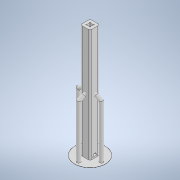
# Autodesk Inventor part: 130mm Rod Template
Saved by Autodesk Inventor 2022 (Build 260153000, 153)
## iProperties
Created: 2022-06-07
Part Number: 130mm Rod Template
Material: Generic
Document SubType Name: Modeling
Designer: Nick
Density: 1 g/cm^3
Appearance: Default
Author: Nick
Autodesk Inventor part; units mm, degrees
ref_plane "YZ Plane" through (0, 0, 0) normal (1, 0, 0) x (0, 1, 0)
ref_plane "XZ Plane" through (0, 0, 0) normal (0, 1, 0) x (-1, 0, 0)
ref_plane "XY Plane" through (0, 0, 0) normal (0, 0, 1) x (1, 0, 0)
sketch "Sketch1" plane through (0, 0, 0) normal (0, 1, 0) x (-1, 0, 0)
  circle A0 centre (0, 0) radius 2
  arc A1 (2.5, 2.179449) -> (2.5, -2.179449) centre (7, 0) ccw
  arc A2 (2.179449, -2.5) -> (-2.179449, -2.5) centre (0, -7) ccw
  arc A3 (-2.5, -2.179449) -> (-2.5, 2.179449) centre (-7, 0) ccw
  arc A4 (-2.179449, 2.5) -> (2.179449, 2.5) centre (0, 7) ccw
  line L0 (2.5, 2.5) -> (-2.5, 2.5)
  line L1 (-2.5, 2.5) -> (-2.5, -2.5)
  line L2 (-2.5, -2.5) -> (2.5, -2.5)
  line L3 (2.5, -2.5) -> (2.5, 2.5)
  line L4 (-5.5, -5.5) -> (-5.5, 5.5)
  line L5 (-5.5, 5.5) -> (5.5, 5.5)
  line L6 (5.5, 5.5) -> (5.5, -5.5)
  line L7 (5.5, -5.5) -> (-5.5, -5.5)
  point P0 (2.5, 0)
  point P1 (0, -2.5)
  dimension "d0" = 4
  dimension "d1" = 5
  dimension "d2" = 5
  dimension "d3" = 3
  constraints: 16 end point, 8 point on circle, 8 point on line, 5 centre point, 4 parallel, 4 tangent, 3 equal radius, 3 horizontal alignment, 3 perpendicular, 3 vertical alignment, 2 midpoint, 1 coincident, 1 horizontal, 3 other
  measures "d0" diameter of A0
  measures "d1" distance of L0.start L0.end
  measures "d2" radius of A4
  measures "d3" distance between parallel lines of L1 L4
extrude "Extrusion1" add sketch "Sketch1" along normal blind 127 contours A1 L3 | A4 L0 | A2 L2 | A3 L1 | L4 L5 L6 L7
sketch "Sketch2" plane through (5.5, 0, -5.5) normal (0, 0, -1) x (-1, 0, 0)
  line L0 (11, 127) -> (11, 0) construction
  line L1 (11, 0) -> (0, 0) construction
  line L2 (0, 0) -> (0, 127) construction
  line L3 (0, 127) -> (11, 127) construction
  line L4 (0, 0) -> (0, 127)
  line L5 (0, 127) -> (11, 127)
  line L6 (11, 0) -> (11, 127)
  line L7 (0, 0) -> (11, 0)
  line L8 (2.45, 73.51013) -> (2.45, 76.485981)
  line L9 (2.45, 76.485981) -> (3.072853, 76.485981)
  line L10 (3.072853, 76.485981) -> (3.072853, 75.378688)
  line L11 (3.072853, 75.378688) -> (7.16094, 75.378688)
  line L12 (7.16094, 75.378688) -> (7.16094, 76.485981)
  line L13 (7.16094, 76.485981) -> (7.71953, 76.485981)
  spline S0 degree 2 poles (7.71953, 76.485981) (7.71953, 75.858185) (8.075446, 75.264993) (8.569773, 75.225446) knots 0 0 0 1 2 2 2
  line L14 (8.569773, 75.225446) -> (8.569773, 74.592707)
  line L15 (8.569773, 74.592707) -> (3.072853, 74.592707)
  line L16 (3.072853, 74.592707) -> (3.072853, 73.51013)
  line L17 (3.072853, 73.51013) -> (2.45, 73.51013)
  spline S1 degree 2 poles (7.971637, 70.741897) (7.971637, 70.964344) (7.862885, 71.404296) (7.778849, 71.616856) knots 0 0 0 1 2 2 2
  spline S2 degree 2 poles (7.778849, 71.616856) (7.694814, 71.814587) (7.516856, 72.10624) (7.437764, 72.219936) knots 0 0 0 1 2 2 2
  line L18 (7.437764, 72.219936) -> (7.437764, 72.269368)
  line L19 (7.437764, 72.269368) -> (8.302836, 72.269368)
  spline S3 degree 2 poles (8.302836, 72.269368) (8.446191, 72.002432) (8.678525, 71.087926) (8.678525, 70.677634) knots 0 0 0 1 2 2 2
  spline S4 degree 2 poles (8.678525, 70.677634) (8.678525, 70.262399) (8.510454, 69.64449) (8.332496, 69.392383) knots 0 0 0 1 2 2 2
  spline S5 degree 2 poles (8.332496, 69.392383) (8.139708, 69.125446) (7.581118, 68.848623) (7.20543, 68.848623) knots 0 0 0 1 2 2 2
  spline S6 degree 2 poles (7.20543, 68.848623) (6.701216, 68.848623) (5.939951, 69.511022) (5.841086, 69.975689) knots 0 0 0 1 2 2 2
  line L20 (5.841086, 69.975689) -> (5.781767, 69.975689)
  spline S7 degree 2 poles (5.781767, 69.975689) (5.742221, 69.782902) (5.564263, 69.34295) (5.386305, 69.155106) knots 0 0 0 1 2 2 2
  spline S8 degree 2 poles (5.386305, 69.155106) (5.21329, 68.967261) (4.659644, 68.729984) (4.259238, 68.729984) knots 0 0 0 1 2 2 2
  spline S9 degree 2 poles (4.259238, 68.729984) (3.848947, 68.729984) (3.151945, 69.011751) (2.885008, 69.268801) knots 0 0 0 1 2 2 2
  spline S10 degree 2 poles (2.885008, 69.268801) (2.608185, 69.535738) (2.321475, 70.292059) (2.321475, 70.771556) knots 0 0 0 1 2 2 2
  spline S11 degree 2 poles (2.321475, 70.771556) (2.321475, 71.231281) (2.543922, 72.130957) (2.697164, 72.43744) knots 0 0 0 1 2 2 2
  line L21 (2.697164, 72.43744) -> (3.562237, 72.43744)
  line L22 (3.562237, 72.43744) -> (3.562237, 72.37812)
  spline S12 degree 2 poles (3.562237, 72.37812) (3.374392, 72.12107) (3.028363, 71.251054) (3.028363, 70.820989) knots 0 0 0 1 2 2 2
  spline S13 degree 2 poles (3.028363, 70.820989) (3.028363, 70.568882) (3.186548, 70.064668) (3.369449, 69.896597) knots 0 0 0 1 2 2 2
  spline S14 degree 2 poles (3.369449, 69.896597) (3.55235, 69.733469) (3.987358, 69.560454) (4.318558, 69.560454) knots 0 0 0 1 2 2 2
  spline S15 degree 2 poles (4.318558, 69.560454) (4.649757, 69.560454) (5.079822, 69.753242) (5.203404, 69.926257) knots 0 0 0 1 2 2 2
  spline S16 degree 2 poles (5.203404, 69.926257) (5.326986, 70.099271) (5.420908, 70.568882) (5.420908, 70.845706) knots 0 0 0 1 2 2 2
  line L23 (5.420908, 70.845706) -> (5.420908, 71.191735)
  line L24 (5.420908, 71.191735) -> (6.098136, 71.191735)
  line L25 (6.098136, 71.191735) -> (6.098136, 70.919855)
  spline S17 degree 2 poles (6.098136, 70.919855) (6.098136, 70.371151) (6.622123, 69.679093) (7.121394, 69.679093) knots 0 0 0 1 2 2 2
  spline S18 degree 2 poles (7.121394, 69.679093) (7.353728, 69.679093) (7.684927, 69.857051) (7.783793, 70.000406) knots 0 0 0 1 2 2 2
  spline S19 degree 2 poles (7.783793, 70.000406) (7.887601, 70.153647) (7.971637, 70.529336) (7.971637, 70.741897) knots 0 0 0 1 2 2 2
  spline S20 degree 2 poles (5.5, 64.014101) (3.858833, 64.014101) (2.321475, 64.968153) (2.321475, 65.961751) knots 0 0 0 1 2 2 2
  spline S21 degree 2 poles (2.321475, 65.961751) (2.321475, 66.970179) (3.888493, 67.914344) (5.495057, 67.914344) knots 0 0 0 1 2 2 2
  spline S22 degree 2 poles (5.495057, 67.914344) (7.14611, 67.914344) (8.673582, 66.960292) (8.673582, 65.961751) knots 0 0 0 1 2 2 2
  spline S23 degree 2 poles (8.673582, 65.961751) (8.673582, 64.958266) (7.091734, 64.014101) (5.5, 64.014101) knots 0 0 0 1 2 2 2
  spline S24 degree 2 poles (3.641329, 65.062075) (3.942869, 64.943436) (4.872204, 64.844571) (5.5, 64.844571) knots 0 0 0 1 2 2 2
  spline S25 degree 2 poles (5.5, 64.844571) (6.127796, 64.844571) (7.052188, 64.943436) (7.363614, 65.067018) knots 0 0 0 1 2 2 2
  spline S26 degree 2 poles (7.363614, 65.067018) (7.675041, 65.1906) (7.996353, 65.620665) (7.996353, 65.961751) knots 0 0 0 1 2 2 2
  spline S27 degree 2 poles (7.996353, 65.961751) (7.996353, 66.302837) (7.675041, 66.742788) (7.353728, 66.871313) knots 0 0 0 1 2 2 2
  spline S28 degree 2 poles (7.353728, 66.871313) (7.042302, 66.994895) (6.093193, 67.083874) (5.495057, 67.083874) knots 0 0 0 1 2 2 2
  spline S29 degree 2 poles (5.495057, 67.083874) (4.852431, 67.083874) (3.992302, 67.004782) (3.656159, 66.876257) knots 0 0 0 1 2 2 2
  spline S30 degree 2 poles (3.656159, 66.876257) (3.339789, 66.757618) (2.998703, 66.317667) (2.998703, 65.961751) knots 0 0 0 1 2 2 2
  spline S31 degree 2 poles (2.998703, 65.961751) (2.998703, 65.625608) (3.320016, 65.185657) (3.641329, 65.062075) knots 0 0 0 1 2 2 2
  line L26 (2.45, 57.928931) -> (5.099595, 57.928931)
  spline S32 degree 2 poles (5.099595, 57.928931) (5.415964, 57.928931) (5.954781, 57.978363) (6.10308, 58.057456) knots 0 0 0 1 2 2 2
  spline S33 degree 2 poles (6.10308, 58.057456) (6.266208, 58.136548) (6.424392, 58.438088) (6.424392, 58.700081) knots 0 0 0 1 2 2 2
  spline S34 degree 2 poles (6.424392, 58.700081) (6.424392, 58.937358) (6.132739, 59.481119) (5.855916, 59.767828) knots 0 0 0 1 2 2 2
  spline S35 degree 2 poles (5.855916, 59.767828) (5.78671, 59.762885) (5.593922, 59.752999) (5.465397, 59.752999) knots 0 0 0 1 2 2 2
  line L27 (5.465397, 59.752999) -> (2.45, 59.752999)
  line L28 (2.45, 59.752999) -> (2.45, 60.524149)
  line L29 (2.45, 60.524149) -> (5.099595, 60.524149)
  spline S36 degree 2 poles (5.099595, 60.524149) (5.415964, 60.524149) (5.954781, 60.573582) (6.10308, 60.652675) knots 0 0 0 1 2 2 2
  spline S37 degree 2 poles (6.10308, 60.652675) (6.266208, 60.731767) (6.424392, 61.033307) (6.424392, 61.2953) knots 0 0 0 1 2 2 2
  spline S38 degree 2 poles (6.424392, 61.2953) (6.424392, 61.542464) (6.112966, 62.091167) (5.870746, 62.348218) knots 0 0 0 1 2 2 2
  line L30 (5.870746, 62.348218) -> (2.45, 62.348218)
  line L31 (2.45, 62.348218) -> (2.45, 63.119368)
  line L32 (2.45, 63.119368) -> (7.027472, 63.119368)
  line L33 (7.027472, 63.119368) -> (7.027472, 62.348218)
  line L34 (7.027472, 62.348218) -> (6.523258, 62.348218)
  spline S39 degree 2 poles (6.523258, 62.348218) (6.824798, 62.046678) (7.155997, 61.453485) (7.155997, 61.097569) knots 0 0 0 1 2 2 2
  spline S40 degree 2 poles (7.155997, 61.097569) (7.155997, 60.692221) (6.785251, 60.064425) (6.365073, 59.901297) knots 0 0 0 1 2 2 2
  spline S41 degree 2 poles (6.365073, 59.901297) (6.755592, 59.550324) (7.155997, 58.887926) (7.155997, 58.50235) knots 0 0 0 1 2 2 2
  spline S42 degree 2 poles (7.155997, 58.50235) (7.155997, 58.205754) (6.973096, 57.721313) (6.765478, 57.543355) knots 0 0 0 1 2 2 2
  spline S43 degree 2 poles (6.765478, 57.543355) (6.557861, 57.360454) (5.935008, 57.15778) (5.465397, 57.15778) knots 0 0 0 1 2 2 2
  line L35 (5.465397, 57.15778) -> (2.45, 57.15778)
  line L36 (2.45, 57.15778) -> (2.45, 57.928931)
  line L37 (2.45, 50.884765) -> (5.099595, 50.884765)
  spline S44 degree 2 poles (5.099595, 50.884765) (5.415964, 50.884765) (5.954781, 50.934198) (6.10308, 51.01329) knots 0 0 0 1 2 2 2
  spline S45 degree 2 poles (6.10308, 51.01329) (6.266208, 51.092383) (6.424392, 51.393922) (6.424392, 51.655916) knots 0 0 0 1 2 2 2
  spline S46 degree 2 poles (6.424392, 51.655916) (6.424392, 51.893193) (6.132739, 52.436953) (5.855916, 52.723663) knots 0 0 0 1 2 2 2
  spline S47 degree 2 poles (5.855916, 52.723663) (5.78671, 52.71872) (5.593922, 52.708833) (5.465397, 52.708833) knots 0 0 0 1 2 2 2
  line L38 (5.465397, 52.708833) -> (2.45, 52.708833)
  line L39 (2.45, 52.708833) -> (2.45, 53.479984)
  line L40 (2.45, 53.479984) -> (5.099595, 53.479984)
  spline S48 degree 2 poles (5.099595, 53.479984) (5.415964, 53.479984) (5.954781, 53.529417) (6.10308, 53.608509) knots 0 0 0 1 2 2 2
  spline S49 degree 2 poles (6.10308, 53.608509) (6.266208, 53.687601) (6.424392, 53.989141) (6.424392, 54.251135) knots 0 0 0 1 2 2 2
  spline S50 degree 2 poles (6.424392, 54.251135) (6.424392, 54.498298) (6.112966, 55.047002) (5.870746, 55.304052) knots 0 0 0 1 2 2 2
  line L41 (5.870746, 55.304052) -> (2.45, 55.304052)
  line L42 (2.45, 55.304052) -> (2.45, 56.075203)
  line L43 (2.45, 56.075203) -> (7.027472, 56.075203)
  line L44 (7.027472, 56.075203) -> (7.027472, 55.304052)
  line L45 (7.027472, 55.304052) -> (6.523258, 55.304052)
  spline S51 degree 2 poles (6.523258, 55.304052) (6.824798, 55.002512) (7.155997, 54.409319) (7.155997, 54.053404) knots 0 0 0 1 2 2 2
  spline S52 degree 2 poles (7.155997, 54.053404) (7.155997, 53.648055) (6.785251, 53.020259) (6.365073, 52.857131) knots 0 0 0 1 2 2 2
  spline S53 degree 2 poles (6.365073, 52.857131) (6.755592, 52.506159) (7.155997, 51.84376) (7.155997, 51.458185) knots 0 0 0 1 2 2 2
  spline S54 degree 2 poles (7.155997, 51.458185) (7.155997, 51.161588) (6.973096, 50.677148) (6.765478, 50.49919) knots 0 0 0 1 2 2 2
  spline S55 degree 2 poles (6.765478, 50.49919) (6.557861, 50.316289) (5.935008, 50.113614) (5.465397, 50.113614) knots 0 0 0 1 2 2 2
  line L46 (5.465397, 50.113614) -> (2.45, 50.113614)
  line L47 (2.45, 50.113614) -> (2.45, 50.884765)
  point P0 (5.5, 0)
  dimension "d0" = 4
  dimension "d1" = 5
  dimension "d2" = 5
  dimension "d3" = 3
  constraints: 4 collinear, 1 vertical, 2 other
emboss "Emboss1" sketch "Sketch2" operation cut depth 0.2 direction (0, 0, 1) contours L8 L9 L10 L11 L12 L13 S0 L14 L15 L16 L17 | S1 S2 L18 L19 S3 S4 S5 S6 L20 S7 S8 S9 S10 S11 L21 L22 S12 S13 S14 S15 S16 L23 L24 L25 S17 S18 S19 | S20 S21 S22 S23 | L26 S32 S33 S34 S35 L27 L28 L29 S36 S37 S38 L30 L31 L32 L33 L34 S39 S40 S41 S42 S43 L35 L36 | L37 S44 S45 S46 S47 L38 L39 L40 S48 S49 S50 L41 L42 L43 L44 L45 S51 S52 S53 S54 S55 L46 L47
fillet "Fillet1" radius 2 4 edges at (-5.5, 63.5, 5.5) (-5.5, 63.5, -5.5) (5.5, 63.5, -5.5) (5.5, 63.5, 5.5)
sketch "Sketch3" plane through (0, 0, 0) normal (0, -1, 0) x (1, 0, 0)
  arc A0 (5.5, 3.5) -> (3.5, 5.5) centre (3.5, 3.5) ccw
  line L0 (-3.5, 5.5) -> (3.5, 5.5)
  arc A1 (-3.5, 5.5) -> (-5.5, 3.5) centre (-3.5, 3.5) ccw
  line L1 (-5.5, -3.5) -> (-5.5, 3.5)
  arc A2 (-5.5, -3.5) -> (-3.5, -5.5) centre (-3.5, -3.5) ccw
  line L2 (3.5, -5.5) -> (-3.5, -5.5)
  arc A3 (3.5, -5.5) -> (5.5, -3.5) centre (3.5, -3.5) ccw
  line L3 (5.5, 3.5) -> (5.5, -3.5)
  arc A4 (-2.5, -2.179449) -> (-2.5, 2.179449) centre (-7, 0) ccw
  line L4 (-2.5, 2.5) -> (-2.5, 2.179449)
  line L5 (-2.179449, 2.5) -> (-2.5, 2.5)
  arc A5 (-2.179449, 2.5) -> (2.179449, 2.5) centre (0, 7) ccw
  line L6 (2.5, 2.5) -> (2.179449, 2.5)
  line L7 (2.5, 2.179449) -> (2.5, 2.5)
  arc A6 (2.5, 2.179449) -> (2.5, -2.179449) centre (7, 0) ccw
  line L8 (2.5, -2.5) -> (2.5, -2.179449)
  line L9 (2.179449, -2.5) -> (2.5, -2.5)
  arc A7 (2.179449, -2.5) -> (-2.179449, -2.5) centre (0, -7) ccw
  line L10 (-2.5, -2.5) -> (-2.179449, -2.5)
  line L11 (-2.5, -2.179449) -> (-2.5, -2.5)
  point P0 (0, 0)
extrude "Extrusion2" add sketch "Sketch3" along normal blind 2 contours L3 A3 L2 A2 L1 A1 L0 A0 | A4 L4 L5 A5 L6 L7 A6 L8 L9 A7 L10 L11
sketch "Sketch4" plane through (5.5, 127, 3.5) normal (1, 0, 0) x (0, 0, -1)
  line L0 (5.679449, -127) -> (1.320551, -127)
  line L1 (6, -124) -> (1, -124)
  line L2 (1, -124) -> (1, -127)
  line L3 (1, -127) -> (6, -127)
  line L4 (6, -127) -> (6, -124)
  line L5 (6, -127) -> (4.267949, -124)
  line L6 (1, -127) -> (2.732051, -124)
  point P0 (3.5, -127)
  point P1 (1.320551, -127)
  dimension "d17" = 5
  dimension "d18" = 3
  dimension "d19" = 60
  dimension "d20" = 60
  constraints: 12 end point, 2 midpoint, 2 parallel, 2 point on line, 1 horizontal, 1 perpendicular
  measures "d17" distance of L3.end L2.end
  measures "d18" distance of L2.end L1.end
  measures "d19" angle of L3 L6
  measures "d20" angle of L3 L5
extrude "Extrusion3" cut sketch "Sketch4" against normal through all contours L0 L3 L6 L1 L5
sketch "Sketch5" plane through (0, -2, 0) normal (0, -1, 0) x (1, 0, 0)
  circle A0 centre (0, 0) radius 17.5
  dimension "d21" = 35
  constraints: 1 centre point, 1 coincident
  measures "d21" diameter of A0
extrude "Extrusion4" add sketch "Sketch5" against normal blind 0.2
sketch "Sketch6" plane through (0, -2, 0) normal (0, -1, 0) x (1, 0, 0)
  circle A0 centre (0, 0) radius 0.75
  dimension "d24" = 1.5
  constraints: 1 centre point, 1 coincident
  measures "d24" diameter of A0
extrude "Extrusion5" cut sketch "Sketch6" against normal through all
sketch "Sketch7" plane through (0, -1.8, 0) normal (0, 1, 0) x (1, 0, 0)
  circle A0 centre (13, 0) radius 2
  circle A1 centre (-13, 0) radius 2
  point P0 (0, 0)
  dimension "d27" = 13
  dimension "d28" = 13
  dimension "d29" = 4
  dimension "d30" = 4
  constraints: 2 centre point, 2 horizontal alignment
  measures "d27" distance of point (0, 0) A1.centre
  measures "d28" distance of A0.centre point (0, 0)
  measures "d29" diameter of A1
  measures "d30" diameter of A0
sketch "Sketch8" plane through (0, 0, 0) normal (0, 0, 1) x (1, 0, 0)
  line L0 (5.5, 127) -> (5.5, -1.8)
  line L1 (-5.5, 127) -> (-5.5, -1.8)
  line L2 (5.5, 127) -> (5.5, -1.8)
  line L3 (5.5, 62.6) -> (13, 55.1)
  line L4 (13, -1.8) -> (13, 55.1)
  line L5 (-5.5, 62.6) -> (-13, 58.269873)
  line L6 (-13, 58.269873) -> (-13, -1.8)
  line L7 (-5.5, 62.6) -> (-4.633975, 63.1)
  point P0 (0, 0)
  dimension "d31" = 135
  dimension "d32" = 120
  dimension "d38" = 1
  constraints: 10 end point, 2 midpoint, 2 vertical, 1 collinear
  measures "d31" angle of L4 L3
  measures "d32" angle of L6 L5
  measures "d38" distance of L5.start L7.end
sweep "Sweep1" add profiles "Sketch7" path "Sketch8" separate body path curves L6 L5 L7 contours A1
chamfer "Chamfer1" distance 2 angle 60 1 edges at (-5.634, 64.8321, 0) measured on face at (-5.384, 64.399, 0)
pattern_circular "Circular Pattern1" count 4 over 360 about axis through (0, -2, 0) along (0, 1, 0) of "Sweep1", "Chamfer1" bodies 2 skipped copies 4
body "Solid1"
body "Solid2"
